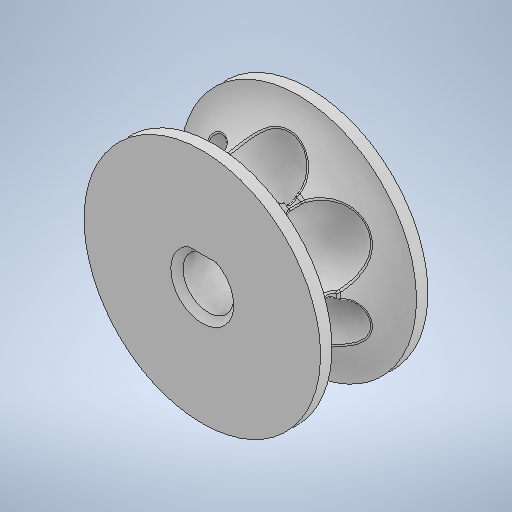
# Autodesk Inventor part: rope_shkif_4.3
Saved by Autodesk Inventor 2025.2 (Build 292293000, 293)
## iProperties
Created: 2025-01-25
Part Number: rope_shkif_4.3
Material: Типовые
Document SubType Name: Modeling
Designer: ignat
Density: 1 g/cm^3
Appearance: По умолчанию
Author: ignat
Autodesk Inventor part; units mm, degrees
ref_plane "YZ Plane" through (0, 0, 0) normal (1, 0, 0) x (0, 1, 0)
ref_plane "XZ Plane" through (0, 0, 0) normal (0, 1, 0) x (-1, 0, 0)
ref_plane "XY Plane" through (0, 0, 0) normal (0, 0, 1) x (1, 0, 0)
sketch "Эскиз1" plane through (0, 0, 0) normal (1, 0, 0) x (0, 1, 0)
  line L0 (0, 0) -> (7.7, 0)
  line L1 (7.7, 7) -> (0, 7)
  line L2 (0, 7) -> (0, 0)
  line L3 (7.7, 0) -> (7.7, 0.75)
  line L4 (7.7, 6.25) -> (7.7, 7)
  arc A0 (4.9756, 3.8741) -> (4.9756, 3.1259) centre (4.95, 3.5) ccw
  arc A1 (7.7, 6.25) -> (4.9756, 3.8741) centre (7.7, 3.5) ccw
  arc A2 (4.9756, 3.1259) -> (7.7, 0.75) centre (7.7, 3.5) ccw
  line L5 (4.2955, 10.0695) -> (0, 10.0695)
  line L6 (0, 10.0695) -> (0, 12.5709)
  line L7 (0, 12.5709) -> (5.5, 12.5709)
  line L8 (4.2955, 8.9677) -> (5.5, 8.9677)
  dimension "d1" = 7
  dimension "d3" = 0.75
  dimension "d9" = 2.75
  dimension "d10" = 2.75
  dimension "d11" = 3.5
  dimension "d33" = 5.5
  dimension "d36" = 2.75
  dimension "d37" = 3.5
  dimension "d39" = 7.7
  dimension "d40" = 2.75
  constraints: 18 end point, 7 perpendicular, 6 point on circle, 3 centre point, 3 horizontal
  measures "d1" distance of L0.end L1.start
  measures "d3" diameter of A0
  measures "d9" radius of A1
  measures "d10" radius of A2
  measures "d11" distance from line of L0 A1.centre
  measures "d33" distance of L6.end L7.end
  measures "d36" distance of A0.centre A1.centre
  measures "d37" distance from line of L0 A0.centre
  measures "d39" distance of L1.start L1.end
  measures "d40" distance from line of L4 A0.centre
revolve "Вращение1" add sketch "Эскиз1" angle 360 about axis through (0, 0, 7) along (0, 0, -1)
sketch "Эскиз2" plane through (0, 0, 7) normal (0, 0, 1) x (1, 0, 0)
  arc A0 (-0.8107, 1.4371) -> (0.8107, 1.4371) centre (0, 0) ccw
  line L0 (-0.8107, 1.4371) -> (0.8107, 1.4371)
  dimension "d5" = 3.3
  constraints: 2 end point, 2 point on circle, 1 centre point, 1 coincident
  measures "d5" diameter of A0
extrude "Выдавливание1" cut sketch "Эскиз2" against normal through all
fillet "Сопряжение1" radius 0.2 2 edges at (0, -4.9756, 3.8741) (0, -4.9756, 3.1259)
ref_plane "РабПлоскость1" through (0, 0, 3.5) normal (0, 0, 1) x (1, 0, 0)
sketch "Эскиз3" plane through (0, 0, 3.5) normal (0, 0, 1) x (1, 0, 0)
  arc A0 (0, 7.3493) -> (0, 2.6493) centre (0, 4.9993) ccw
  circle A1 centre (45.9958, -0.3039) radius 5.5
  circle A2 centre (39.9958, -0.3039) radius 2.35
  circle A3 centre (43.2458, 4.4593) radius 2.35
  circle A4 centre (48.7458, 4.4593) radius 2.35
  circle A5 centre (51.4958, -0.3039) radius 2.35
  circle A6 centre (48.7458, -5.067) radius 2.35
  circle A7 centre (42.9958, -5.5) radius 2.35
  line L0 (0, 7.3493) -> (0, 2.6493)
  circle A8 centre (0, 0) radius 4.9993 projected
  line L1 (0, 5.4821) -> (0, 4.9993)
  point P0 (0, 4.0934)
  dimension "d13" = 4.7
  dimension "d16" = 11
  dimension "d19" = 4.7
  dimension "d20" = 4.7
  dimension "d21" = 4.7
  dimension "d22" = 4.7
  dimension "d23" = 4.7
  dimension "d24" = 4.7
  constraints: 8 centre point, 6 point on circle, 4 end point, 1 vertical, 1 vertical alignment, 1 other
  measures "d13" diameter of A0
  measures "d16" diameter of A1
  measures "d19" diameter of A2
  measures "d20" diameter of A3
  measures "d21" diameter of A4
  measures "d22" diameter of A5
  measures "d23" diameter of A6
  measures "d24" diameter of A7
revolve "Вращение2" cut sketch "Эскиз3" angle 360 about axis through (0, 7.3493, 3.5) along (0, -1, 0) picked at (-0.7538, 5.7495) picked at (-0.4352, 4.2144) contours L0 A8 A0 | A8 L0 A0
pattern_circular "Круговой массив1" count 6 over 360 about axis through (0, 0, 7) along (0, 0, -1) of "Вращение2"
fillet "Сопряжение2" radius 0.1 56 edges at (-2.2371, 4.4146, 3.9194) (-2.1664, 4.1178, 3.7288) (-2.1664, 4.1178, 3.2712) (-2.2371, 4.4146, 3.0806) (1.5284, 5.3631, 1.7524) (-1.5285, 5.3631, 1.7524) (2.2371, 4.4146, 3.0806) (2.1456, 4.0407, 3.5) (2.2371, 4.4146, 3.9194) (1.5284, 5.3631, 5.2476) (-1.5284, 5.3631, 5.2476) (2.7046, -4.1447, 3.0806) (2.4265, -3.8785, 3.5) (2.7046, -4.1447, 3.9194) (5.1718, -2.986, 5.6392) (4.9417, -0.2699, 3.9194) (4.6493, -0.1828, 3.7288) (4.6493, -0.1828, 3.2712) (4.9417, -0.2699, 3.0806) (5.1719, -2.9859, 1.3608) (-4.9417, -0.2699, 3.0806) (-4.5721, -0.1622, 3.5) (-4.9417, -0.2699, 3.9194) (-5.1719, -2.9859, 5.6392) (-2.7046, -4.1447, 3.9194) (-2.4829, -3.935, 3.7288) (-2.4829, -3.935, 3.2712) (-2.7046, -4.1447, 3.0806) (-5.1718, -2.986, 1.3608) (-2.7046, 4.1447, 3.0806) (-2.4265, 3.8785, 3.5) (-2.7046, 4.1447, 3.9194) (-5.1718, 2.986, 5.6392) (-4.9417, 0.2699, 3.9194) (-4.6493, 0.1828, 3.7288) (-4.6493, 0.1828, 3.2712) (-4.9417, 0.2699, 3.0806) (-5.1719, 2.9859, 1.3608) (4.9417, 0.2699, 3.0806) (4.5721, 0.1622, 3.5) (4.9417, 0.2699, 3.9194) (5.1719, 2.9859, 5.6392) (2.7046, 4.1447, 3.9194) (2.4829, 3.935, 3.7288) (2.4829, 3.935, 3.2712) (2.7046, 4.1447, 3.0806) (5.1718, 2.986, 1.3608) (-2.2371, -4.4146, 3.0806) (-2.1456, -4.0407, 3.5) (-2.2371, -4.4146, 3.9194) (0, -5.972, 5.6392) (2.2371, -4.4146, 3.9194) (2.1664, -4.1178, 3.7288) (2.1664, -4.1178, 3.2712) (2.2371, -4.4146, 3.0806) (0, -5.972, 1.3608)
chamfer "Фаска1" distance 0.4 angle 45 4 edges at (0, 1.4371, 7) (0, -1.65, 7) (0, -1.65, 0) (0, 1.4371, 0)
